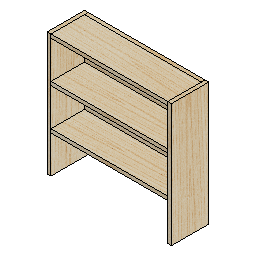
model (Autodesk Fusion 360 design; units mm, degrees)
Autodesk Fusion 360 part; units mm, degrees
sketch "Sketch1" plane through (0, 0, 0) normal (0, 1, 0) x (1, 0, 0) in component "shelf"
  line L0 (400, 0) -> (400, -396)
  line L1 (400, -396) -> (0, -396)
  line L2 (0, -396) -> (0, 0)
  line L3 (0, 0) -> (12, 0)
  line L4 (12, 0) -> (12, -120)
  line L5 (12, -120) -> (388, -120)
  line L6 (388, -120) -> (388, 0)
  line L7 (388, 0) -> (400, 0)
  line L8 (12, -252) -> (388, -252)
  line L9 (388, -252) -> (388, -132)
  line L10 (388, -132) -> (12, -132)
  line L11 (12, -132) -> (12, -252)
  line L12 (12, -120) -> (12, -132)
  line L13 (12, -264) -> (388, -264)
  line L14 (388, -264) -> (388, -384)
  line L15 (388, -384) -> (12, -384)
  line L16 (12, -384) -> (12, -264)
  line L17 (12, -252) -> (12, -264)
  line L18 (12, -384) -> (12, -396)
  line L19 (388, -264) -> (388, -252)
  line L20 (388, -132) -> (388, -120)
  line L21 (388, -384) -> (388, -396)
  dimension "d4" = 120
  dimension "d6" = 12
  dimension "d7" = 400
  dimension "d8" = 396
  constraint vertical L0
  constraint horizontal L1
  constraint vertical L2
  constraint coincident L2.end L3.start
  constraint horizontal L3
  constraint vertical L4
  constraint horizontal L5
  constraint vertical L6
  constraint horizontal L7
  constraint equal L3 L7
  constraint horizontal L8
  constraint vertical L9
  constraint horizontal L10
  constraint vertical L11
  constraint equal L4 L11
  constraint collinear L4 L11
  constraint collinear L6 L9
  constraint equal L3 L12
  constraint horizontal L13
  constraint vertical L14
  constraint horizontal L15
  constraint vertical L16
  constraint collinear L11 L16
  constraint collinear L9 L14
  constraint equal L3 L17
  constraint coincident L1 L18.end
  constraint equal L3 L18
  constraint equal L11 L16
  constraint coincident L1 L21.end
  constraint vertical L21
  constraint vertical L18
  measures "d4" distance of L3 L5
  measures "d6" distance of L2.end L3.end
  measures "d7" distance of L0.end L1.end
  measures "d8" distance of L2.end L1.end
extrude "Extrude1" add sketch "Sketch1" against normal blind 108 from surface at -12 contours L1 L15 L18 L21 | L5 L10 L12 L20 | L8 L13 L17 L19 makes body 1 at (262.6667, -48, 132) makes body 2 at (137.3333, -48, 264) makes body 3 at (262.6667, -48, 396) in component "shelf"
extrude "Extrude2" add sketch "Sketch1" against normal up to surface (120 mm away) separate body contours L0 L1 L6 L7 L9 L14 L19 L20 L21 | L1 L2 L3 L4 L11 L12 L16 L17 L18 makes body 4 at (400, -40, 132) makes body 5 at (0, -40, 264) in component "shelf"
extrude "Extrude3" add sketch "Sketch1" against normal up to surface (12 mm away) separate body contours L1 L15 L18 L21 | L5 L10 L12 L20 | L13 L14 L15 L16 | L8 L9 L10 L11 | L8 L13 L17 L19 makes body 6 in component "shelf"
sketch "Sketch1 (2)" plane through (0, 0, 0) normal (0, 0, 1) x (1, 0, 0) in component "cutlist"
  line L0 (0, 0) -> (0, 100) construction
  line L1 (0, 100) -> (108, 100)
  line L2 (108, 100) -> (108, 476)
  line L3 (108, 476) -> (0, 476)
  line L4 (0, 476) -> (0, 100)
  line L5 (113, 100) -> (221, 100)
  line L6 (221, 100) -> (221, 476)
  line L7 (113, 476) -> (113, 100)
  line L8 (221, 476) -> (113, 476)
  line L9 (226, 100) -> (334, 100)
  line L10 (334, 100) -> (334, 476)
  line L11 (226, 476) -> (226, 100)
  line L12 (334, 476) -> (226, 476)
  line L13 (434, 100) -> (554, 100)
  line L14 (554, 100) -> (554, 496)
  line L15 (554, 496) -> (434, 496)
  line L16 (434, 496) -> (434, 100)
  line L17 (334, 100) -> (434, 100) construction
  line L18 (559, 100) -> (679, 100)
  line L19 (679, 100) -> (679, 496)
  line L20 (559, 496) -> (559, 100)
  line L21 (679, 496) -> (559, 496)
  line L22 (779, 100) -> (1055, 100)
  line L23 (1055, 100) -> (1055, 476)
  line L24 (1055, 476) -> (779, 476)
  line L25 (779, 476) -> (779, 100)
  line L26 (679, 100) -> (779, 100) construction
  dimension "d17" = 100
  dimension "d18" = 376
  dimension "d19" = 108
  dimension "d22" = 113
  dimension "d23" = 0
  dimension "d24" = 396
  dimension "d25" = 120
  dimension "d28" = 125
  dimension "d29" = 0
  dimension "d30" = 276
  dimension "d31" = 334
  dimension "d32" = 245
  constraint coincident L0.start origin
  constraint vertical L0
  constraint horizontal L1
  constraint vertical L2
  constraint horizontal L3
  constraint vertical L4
  constraint horizontal L13
  constraint vertical L14
  constraint horizontal L15
  constraint vertical L16
  constraint collinear L1 L13
  constraint perpendicular L16 L17
  constraint equal L0 L17
  constraint horizontal L22
  constraint vertical L23
  constraint horizontal L24
  constraint vertical L25
  constraint collinear L3 L24
  constraint horizontal L26
  constraint equal L0 L26
  measures "d17" distance of L0.start L0.end
  measures "d18" distance of L0.end L3.end
  measures "d19" distance of L2.end L3.end
  measures "d24" distance of L13.start L15.end
  measures "d25" distance of L14.end L15.end
  measures "d30" distance of L23.end L24.end
  measures "d31" distance of L0.end L9.end
  measures "d32" distance of L15.end L19.end
component "shelf" placed x (1, 0, 0) y (0, 1, 0) z (0, 0, 1) at (0, 0, 0)
component "cutlist" placed x (1, 0, 0) y (0, 1, 0) z (0, 0, 1) at (0, 0, 0)
equation "bottomMinHeight = 120 mm"
equation "maxHeight = 400 mm"
equation "d4 = bottomMinHeight"
equation "plyT = 12 mm"
equation "d6 = plyT"
equation "maxDepth = 120 mm"
equation "d10 = -plyT"
equation "d11 = -maxDepth + plyT"
equation "d18 = 400 mm - 2 * plyT"
equation "d19 = maxDepth - plyT"
equation "d22 = 5 mm + ( maxDepth - plyT )"
equation "d25 = maxDepth"
equation "d28 = 5 mm + maxDepth"
